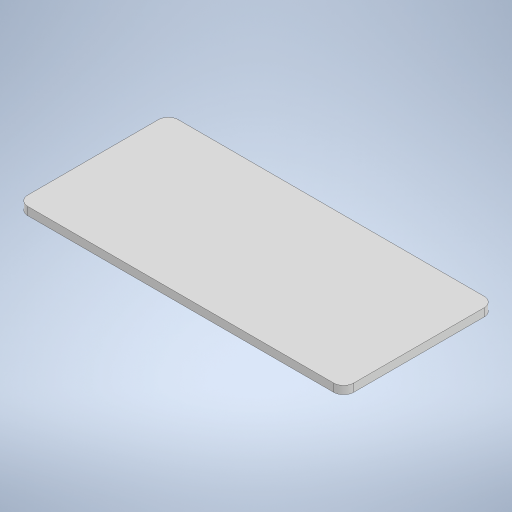
# Autodesk Inventor part: MS_PCB
Saved by Autodesk Inventor 2023 (Build 270158000, 158)
## iProperties
Created: 2024-04-30
Part Number: MS_PCB
Material: Ogólny
Document SubType Name: Modeling
Designer: kamil
Density: 1 g/cm^3
Appearance: Domyślna
Author: kamil
Autodesk Inventor part; units mm, degrees
ref_plane "YZ Plane" through (0, 0, 0) normal (1, 0, 0) x (0, 1, 0)
ref_plane "XZ Plane" through (0, 0, 0) normal (0, 1, 0) x (-1, 0, 0)
ref_plane "XY Plane" through (0, 0, 0) normal (0, 0, 1) x (1, 0, 0)
sketch "Szkic1" plane through (0, 0, 0) normal (0, 1, 0) x (-1, 0, 0)
  line L0 (35.259, 49.5664) -> (-29.741, 49.5664)
  line L1 (-29.741, 49.5664) -> (-29.741, 19.5664)
  line L2 (-29.741, 19.5664) -> (35.259, 19.5664)
  line L3 (35.259, 19.5664) -> (35.259, 49.5664)
  point P0 (0, 0)
  dimension "d0" = 65
  dimension "d1" = 30
  constraints: 8 end point, 2 parallel, 1 horizontal, 1 perpendicular
  measures "d0" distance of L2.end L1.end
  measures "d1" distance of L1.end L0.end
extrude "Wyciągnięcie proste1" add sketch "Szkic1" along normal blind 1.6
fillet "Zaokrąglenie1" radius 2 4 edges at (-35.259, 0.8, 19.5664) (-35.259, 0.8, 49.5664) (29.741, 0.8, 49.5664) (29.741, 0.8, 19.5664)
